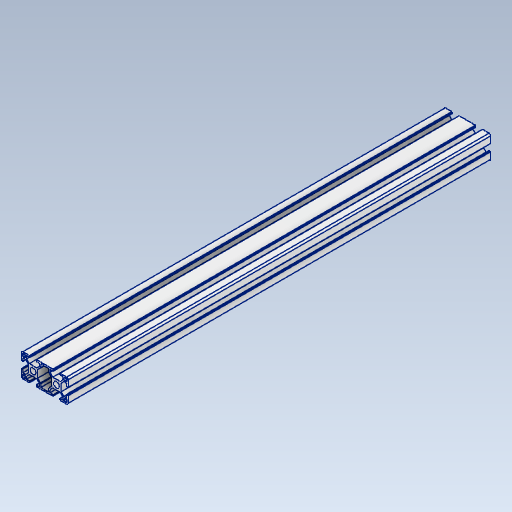
# Autodesk Inventor part: 30x60 aluminum
Saved by Autodesk Inventor 2020.2 (Build 242310000, 310)
## iProperties
Created: 2019-10-30
Part Number: 30x60 aluminum
Material: Aluminum 6061
Document SubType Name: Modeling
Designer: Sunoj
Density: 2.7 g/cm^3
Appearance: Aluminum - Flat
Mass: 819.298 g
Surface Area: 2922.88 cm^2
Volume: 303.444 cm^3
d0: 540.000 mm
Author: Sunoj
Autodesk Inventor part; units mm, degrees
ref_plane "YZ Plane" through (0, 0, 0) normal (1, 0, 0) x (0, 1, 0)
ref_plane "XZ Plane" through (0, 0, 0) normal (0, 1, 0) x (-1, 0, 0)
ref_plane "XY Plane" through (0, 0, 0) normal (0, 0, 1) x (1, 0, 0)
sketch "Sketch1" plane through (0, 0, 0) normal (0, 0, 1) x (1, 0, 0)
  line L0 (-4.1, 13) -> (-4.1, 14)
  line L1 (-4.1, 14) -> (-4.6, 14)
  line L2 (-4.6, 14) -> (-4.6, 15)
  line L3 (-4.6, 14) -> (-4.6, 15)
  line L4 (-4.6, 15) -> (-13, 15)
  arc A0 (-13, 15) -> (-15, 13) centre (-13, 13) ccw
  line L5 (-15, 13) -> (-15, 4.6)
  line L6 (-15, 13) -> (-15, 4.6)
  line L7 (-15, 4.6) -> (-14, 4.6)
  line L8 (-15, 4.6) -> (-14, 4.6)
  line L9 (-14, 4.6) -> (-14, 4.1)
  line L10 (-14, 4.6) -> (-14, 4.1)
  line L11 (-14, 4.1) -> (-13, 4.1)
  line L12 (-13, 4.1) -> (-13, 8.25)
  line L13 (-13, 8.25) -> (-9.5, 8.25)
  line L14 (-13, 8.25) -> (-9.5, 8.25)
  line L15 (-9.5, 8.25) -> (-6, 4.75)
  line L16 (-6, 4.75) -> (-6, -4.75)
  line L17 (-6, 4.75) -> (-6, -4.75)
  line L18 (-6, -4.75) -> (-9.5, -8.25)
  line L19 (-14, -4.1) -> (-13, -4.1)
  line L20 (-13, -4.1) -> (-14, -4.1)
  line L21 (-14, -4.6) -> (-14, -4.1)
  line L22 (-14, -4.1) -> (-14, -4.6)
  line L23 (-15, -4.6) -> (-14, -4.6)
  line L24 (-14, -4.6) -> (-15, -4.6)
  line L25 (-8.25, 13) -> (-4.1, 13)
  line L26 (-4.1, 13) -> (-8.25, 13)
  line L27 (-8.25, 9.5) -> (-8.25, 13)
  line L28 (-8.25, 13) -> (-8.25, 9.5)
  line L29 (-4.75, 6) -> (-8.25, 9.5)
  line L30 (-8.25, 9.5) -> (-4.75, 6)
  line L31 (4.75, 6) -> (-4.75, 6)
  line L32 (-4.75, 6) -> (4.75, 6)
  line L33 (4.75, 6) -> (8.25, 9.5)
  line L34 (8.25, 13) -> (8.25, 9.5)
  line L35 (8.25, 9.5) -> (8.25, 13)
  line L36 (8.25, 13) -> (4.1, 13)
  line L37 (4.1, 13) -> (4.1, 14)
  line L38 (4.6, 14) -> (4.1, 14)
  line L39 (4.1, 14) -> (4.6, 14)
  line L40 (4.6, 15) -> (4.6, 14)
  line L41 (4.6, 14) -> (4.6, 15)
  line L42 (4.6, 15) -> (13.08, 15)
  line L43 (6, 4.75) -> (9.5, 8.25)
  line L44 (9.5, 8.25) -> (6, 4.75)
  line L45 (6, 4.75) -> (6, -4.75)
  circle A1 centre (0, 0) radius 3.75
  line L46 (0, 0) -> (7.2487, 0)
  line L47 (-9.5, -8.25) -> (-6, -4.75)
  line L48 (-8.25, -9.5) -> (-4.75, -6)
  line L49 (-4.75, -6) -> (-8.25, -9.5)
  line L50 (-4.1, -13) -> (-4.1, -14)
  line L51 (-4.1, -14) -> (-4.6, -14)
  line L52 (-8.25, -13) -> (-4.1, -13)
  line L53 (-4.1, -13) -> (-8.25, -13)
  line L54 (-8.25, -9.5) -> (-8.25, -13)
  line L55 (-8.25, -13) -> (-8.25, -9.5)
  line L56 (-13, -8.25) -> (-9.5, -8.25)
  line L57 (-13, -4.1) -> (-13, -8.25)
  line L58 (-4.6, -14) -> (-4.6, -15)
  line L59 (-4.6, -14) -> (-4.6, -15)
  line L60 (-4.6, -15) -> (-13, -15)
  line L61 (-14, -4.6) -> (-14, -4.1)
  line L62 (-14, -4.6) -> (-14, -4.1)
  line L63 (-14, -4.1) -> (-13, -4.1)
  line L64 (-15, -4.6) -> (-14, -4.6)
  line L65 (-15, -4.6) -> (-14, -4.6)
  line L66 (-15, -13) -> (-15, -4.6)
  line L67 (-15, -13) -> (-15, -4.6)
  arc A2 (-15, -13) -> (-13, -15) centre (-13, -13) ccw
  line L68 (-13, -8.25) -> (-9.5, -8.25)
  line L69 (8.25, -13) -> (8.25, -9.5)
  line L70 (8.25, -9.5) -> (8.25, -13)
  line L71 (4.75, -6) -> (8.25, -9.5)
  line L72 (6, -4.75) -> (9.5, -8.25)
  line L73 (9.5, -8.25) -> (6, -4.75)
  line L74 (8.25, -13) -> (4.1, -13)
  line L75 (4.1, -13) -> (4.1, -14)
  line L76 (4.6, -14) -> (4.1, -14)
  line L77 (4.1, -14) -> (4.6, -14)
  line L78 (4.6, -15) -> (4.6, -14)
  line L79 (4.6, -14) -> (4.6, -15)
  line L80 (4.6, -15) -> (13.08, -15)
  line L81 (4.75, -6) -> (-4.75, -6)
  line L82 (-4.75, -6) -> (4.75, -6)
  circle A3 centre (0, 0) radius 3.75
  line L83 (-12.5, 13.5) -> (-10.7, 13.5)
  line L84 (-12.5, 13.5) -> (-10.7, 13.5)
  line L85 (-9.7, 12.5) -> (-9.7, 10.7)
  line L86 (-9.7, 12.5) -> (-9.7, 10.7)
  line L87 (-10.7, 9.7) -> (-12.5, 9.7)
  line L88 (-10.7, 9.7) -> (-12.5, 9.7)
  line L89 (-13.5, 12.5) -> (-13.5, 10.7)
  line L90 (-13.5, 10.7) -> (-13.5, 12.5)
  line L91 (-13.5, 12.5) -> (-13.5, 10.7)
  arc A4 (-12.5, 13.5) -> (-13.5, 12.5) centre (-12.5, 12.5) ccw
  arc A5 (-13.5, 10.7) -> (-12.5, 9.7) centre (-12.5, 10.7) ccw
  arc A6 (-13.5, 10.7) -> (-12.5, 9.7) centre (-12.5, 10.7) ccw
  arc A7 (-10.7, 9.7) -> (-9.7, 10.7) centre (-10.7, 10.7) ccw
  arc A8 (-9.7, 12.5) -> (-10.7, 13.5) centre (-10.7, 12.5) ccw
  arc A9 (-9.7, 12.5) -> (-10.7, 13.5) centre (-10.7, 12.5) ccw
  line L92 (0, 0) -> (0, 6.5)
  arc A10 (-13.5, -12.5) -> (-12.5, -13.5) centre (-12.5, -12.5) ccw
  line L93 (-9.7, -12.5) -> (-9.7, -10.7)
  line L94 (-9.7, -12.5) -> (-9.7, -10.7)
  line L95 (-10.7, -9.7) -> (-12.5, -9.7)
  line L96 (-10.7, -9.7) -> (-12.5, -9.7)
  line L97 (-13.5, -12.5) -> (-13.5, -10.7)
  line L98 (-13.5, -10.7) -> (-13.5, -12.5)
  line L99 (-13.5, -12.5) -> (-13.5, -10.7)
  arc A11 (-12.5, -9.7) -> (-13.5, -10.7) centre (-12.5, -10.7) ccw
  arc A12 (-12.5, -9.7) -> (-13.5, -10.7) centre (-12.5, -10.7) ccw
  arc A13 (-9.7, -10.7) -> (-10.7, -9.7) centre (-10.7, -10.7) ccw
  line L100 (-12.5, -13.5) -> (-10.7, -13.5)
  line L101 (-12.5, -13.5) -> (-10.7, -13.5)
  arc A14 (-10.7, -13.5) -> (-9.7, -12.5) centre (-10.7, -12.5) ccw
  arc A15 (-10.7, -13.5) -> (-9.7, -12.5) centre (-10.7, -12.5) ccw
  line L102 (34.1, 13) -> (34.1, 14)
  line L103 (34.1, 14) -> (34.6, 14)
  line L104 (34.6, 14) -> (34.6, 15)
  line L105 (34.6, 14) -> (34.6, 15)
  line L106 (34.6, 15) -> (43, 15)
  arc A16 (45, 13) -> (43, 15) centre (43, 13) ccw
  line L107 (45, 13) -> (45, 4.6)
  line L108 (45, 13) -> (45, 4.6)
  line L109 (45, 4.6) -> (44, 4.6)
  line L110 (45, 4.6) -> (44, 4.6)
  line L111 (44, 4.6) -> (44, 4.1)
  line L112 (44, 4.6) -> (44, 4.1)
  line L113 (44, 4.1) -> (43, 4.1)
  line L114 (43, 4.1) -> (43, 8.25)
  line L115 (43, 8.25) -> (39.5, 8.25)
  line L116 (43, 8.25) -> (39.5, 8.25)
  line L117 (39.5, 8.25) -> (36, 4.75)
  line L118 (36, 4.75) -> (36, -4.75)
  line L119 (36, 4.75) -> (36, -4.75)
  line L120 (36, -4.75) -> (39.5, -8.25)
  line L121 (44, -4.1) -> (43, -4.1)
  line L122 (43, -4.1) -> (44, -4.1)
  line L123 (44, -4.6) -> (44, -4.1)
  line L124 (44, -4.1) -> (44, -4.6)
  line L125 (45, -4.6) -> (44, -4.6)
  line L126 (44, -4.6) -> (45, -4.6)
  line L127 (38.25, 13) -> (34.1, 13)
  line L128 (34.1, 13) -> (38.25, 13)
  line L129 (38.25, 9.5) -> (38.25, 13)
  line L130 (38.25, 13) -> (38.25, 9.5)
  line L131 (34.75, 6) -> (38.25, 9.5)
  line L132 (38.25, 9.5) -> (34.75, 6)
  line L133 (25.25, 6) -> (34.75, 6)
  line L134 (34.75, 6) -> (25.25, 6)
  line L135 (25.25, 6) -> (21.75, 9.5)
  line L136 (21.75, 13) -> (21.75, 9.5)
  line L137 (21.75, 9.5) -> (21.75, 13)
  line L138 (21.75, 13) -> (25.9, 13)
  line L139 (25.9, 13) -> (25.9, 14)
  line L140 (25.4, 14) -> (25.9, 14)
  line L141 (25.9, 14) -> (25.4, 14)
  line L142 (25.4, 15) -> (25.4, 14)
  line L143 (25.4, 14) -> (25.4, 15)
  line L144 (25.4, 15) -> (16.92, 15)
  line L145 (24, 4.75) -> (20.5, 8.25)
  line L146 (20.5, 8.25) -> (24, 4.75)
  line L147 (24, 4.75) -> (24, -4.75)
  circle A17 centre (30, 0) radius 3.75
  line L148 (30, 0) -> (22.7513, 0)
  line L149 (39.5, -8.25) -> (36, -4.75)
  line L150 (38.25, -9.5) -> (34.75, -6)
  line L151 (34.75, -6) -> (38.25, -9.5)
  line L152 (34.1, -13) -> (34.1, -14)
  line L153 (34.1, -14) -> (34.6, -14)
  line L154 (38.25, -13) -> (34.1, -13)
  line L155 (34.1, -13) -> (38.25, -13)
  line L156 (38.25, -9.5) -> (38.25, -13)
  line L157 (38.25, -13) -> (38.25, -9.5)
  line L158 (43, -8.25) -> (39.5, -8.25)
  line L159 (43, -4.1) -> (43, -8.25)
  line L160 (34.6, -14) -> (34.6, -15)
  line L161 (34.6, -14) -> (34.6, -15)
  line L162 (34.6, -15) -> (43, -15)
  line L163 (44, -4.6) -> (44, -4.1)
  line L164 (44, -4.6) -> (44, -4.1)
  line L165 (44, -4.1) -> (43, -4.1)
  line L166 (45, -4.6) -> (44, -4.6)
  line L167 (45, -4.6) -> (44, -4.6)
  line L168 (45, -13) -> (45, -4.6)
  line L169 (45, -13) -> (45, -4.6)
  arc A18 (43, -15) -> (45, -13) centre (43, -13) ccw
  line L170 (43, -8.25) -> (39.5, -8.25)
  line L171 (21.75, -13) -> (21.75, -9.5)
  line L172 (21.75, -9.5) -> (21.75, -13)
  line L173 (25.25, -6) -> (21.75, -9.5)
  line L174 (24, -4.75) -> (20.5, -8.25)
  line L175 (20.5, -8.25) -> (24, -4.75)
  line L176 (21.75, -13) -> (25.9, -13)
  line L177 (25.9, -13) -> (25.9, -14)
  line L178 (25.4, -14) -> (25.9, -14)
  line L179 (25.9, -14) -> (25.4, -14)
  line L180 (25.4, -15) -> (25.4, -14)
  line L181 (25.4, -14) -> (25.4, -15)
  line L182 (25.4, -15) -> (16.92, -15)
  line L183 (25.25, -6) -> (34.75, -6)
  line L184 (34.75, -6) -> (25.25, -6)
  circle A19 centre (30, 0) radius 3.75
  line L185 (42.5, 13.5) -> (40.7, 13.5)
  line L186 (42.5, 13.5) -> (40.7, 13.5)
  line L187 (39.7, 12.5) -> (39.7, 10.7)
  line L188 (39.7, 12.5) -> (39.7, 10.7)
  line L189 (40.7, 9.7) -> (42.5, 9.7)
  line L190 (40.7, 9.7) -> (42.5, 9.7)
  line L191 (43.5, 12.5) -> (43.5, 10.7)
  line L192 (43.5, 10.7) -> (43.5, 12.5)
  line L193 (43.5, 12.5) -> (43.5, 10.7)
  arc A20 (43.5, 12.5) -> (42.5, 13.5) centre (42.5, 12.5) ccw
  arc A21 (42.5, 9.7) -> (43.5, 10.7) centre (42.5, 10.7) ccw
  arc A22 (42.5, 9.7) -> (43.5, 10.7) centre (42.5, 10.7) ccw
  arc A23 (39.7, 10.7) -> (40.7, 9.7) centre (40.7, 10.7) ccw
  arc A24 (40.7, 13.5) -> (39.7, 12.5) centre (40.7, 12.5) ccw
  arc A25 (40.7, 13.5) -> (39.7, 12.5) centre (40.7, 12.5) ccw
  arc A26 (42.5, -13.5) -> (43.5, -12.5) centre (42.5, -12.5) ccw
  line L194 (39.7, -12.5) -> (39.7, -10.7)
  line L195 (39.7, -12.5) -> (39.7, -10.7)
  line L196 (40.7, -9.7) -> (42.5, -9.7)
  line L197 (40.7, -9.7) -> (42.5, -9.7)
  line L198 (43.5, -12.5) -> (43.5, -10.7)
  line L199 (43.5, -10.7) -> (43.5, -12.5)
  line L200 (43.5, -12.5) -> (43.5, -10.7)
  arc A27 (43.5, -10.7) -> (42.5, -9.7) centre (42.5, -10.7) ccw
  arc A28 (43.5, -10.7) -> (42.5, -9.7) centre (42.5, -10.7) ccw
  arc A29 (40.7, -9.7) -> (39.7, -10.7) centre (40.7, -10.7) ccw
  line L201 (42.5, -13.5) -> (40.7, -13.5)
  line L202 (42.5, -13.5) -> (40.7, -13.5)
  arc A30 (39.7, -12.5) -> (40.7, -13.5) centre (40.7, -12.5) ccw
  arc A31 (39.7, -12.5) -> (40.7, -13.5) centre (40.7, -12.5) ccw
  line L203 (13.08, -15) -> (16.92, -15)
  line L204 (8.25, 11.25) -> (10, 11.25) construction
  line L205 (9.5, 8.25) -> (10, 8.8)
  line L206 (10, 8.8) -> (10, 13)
  line L207 (8.84, 0) -> (15.75, 0) construction
  line L208 (9.5, -8.25) -> (10, -8.8)
  line L209 (10, -8.8) -> (10, -13)
  line L210 (15, 0) -> (15, 3.7523) construction
  line L211 (20, -8.8) -> (20, -13)
  line L212 (20.5, -8.25) -> (20, -8.8)
  line L213 (24, 4.75) -> (20.5, 8.25)
  line L214 (20.5, 8.25) -> (24, 4.75)
  line L215 (20.5, 8.25) -> (20, 8.8)
  line L216 (20, 8.8) -> (20, 13)
  line L217 (10, 13) -> (20, 13)
  line L218 (13.08, 15) -> (16.92, 15)
  line L219 (10, -13) -> (20, -13)
  point P0 (14.7321, -14)
  point P1 (14.7321, 14)
  point P2 (13.5, -10.7)
  point P3 (14.7321, 14)
  point P4 (14.7321, -14)
  point P5 (13.5, -10.7)
  constraints: 440 end point, 64 point on circle, 42 symmetric about line, 32 centre point, 14 perpendicular, 11 collinear, 9 point on line, 7 horizontal, 4 vertical, 3 parallel, 2 coincident, 2 tangent, 1 midpoint, 7 other
extrude "Extrusion1" add sketch "Sketch1" along normal blind 540
body "Solid1"
